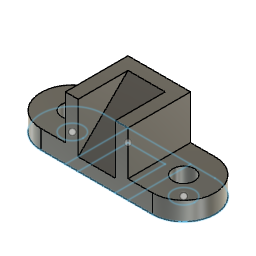
A2 (Autodesk Fusion 360 design; units mm, degrees)
Autodesk Fusion 360 part; units mm, degrees
sketch "Sketch1" plane through (0, 0, 0) normal (0, 0, 1) x (1, 0, 0)
  circle A0 centre (-57, 0.002) radius 11
  circle A1 centre (57, 0.0006) radius 11
  line L0 (57.0004, 32.0006) -> (-56.9996, 32.002)
  line L1 (-57.0004, -31.998) -> (56.9996, -31.9994)
  line L2 (-32, 32.0017) -> (-32.0007, -31.9983)
  line L3 (32.0004, 32.0009) -> (31.9996, -31.9991)
  line L4 (-19.0007, -31.9985) -> (-19.0002, 19.0015)
  line L5 (18.9996, -31.9989) -> (19.0002, 19.0011)
  line L6 (-19.0004, 19.0015) -> (19.0002, 19.0011)
  arc A2 (-56.9996, 32.002) -> (-57.0004, -31.998) centre (-57, 0.002) ccw
  arc A3 (56.9996, -31.9994) -> (57.0004, 32.0006) centre (57, 0.0006) ccw
  dimension "d1" = 22
  dimension "d2" = 57
  dimension "d3" = 22
  dimension "d4" = 57
  dimension "d7" = 114
  dimension "d8" = 64
  dimension "d9" = 32
  dimension "d10" = 32
  dimension "d13" = 51
  constraint tangent L0 A2
  constraint tangent L0 A3
  constraint tangent L1 A3
  constraint tangent L1 A2
  constraint coincident L1 L2.end
  constraint perpendicular L1 L2
  constraint coincident L0 L3.start
  constraint coincident L1 L3.end
  constraint perpendicular L1 L3
  constraint perpendicular L0 L4
  constraint perpendicular L0 L5
  constraint perpendicular L5 L6
  constraint coincident L6 L4.end
  constraint concentric A0 A2
  constraint concentric A1 A3
  constraint perpendicular L0 L2
  constraint coincident L0 L2.start
  constraint coincident L1 L4.start
  constraint coincident L1 L5.start
  measures "d1" diameter of A0
  measures "d2" horizontal distance of origin A0.centre
  measures "d3" diameter of A1
  measures "d4" distance of origin A1.centre
  measures "d7" horizontal distance of L0.start L0.end
  measures "d8" vertical distance of L0.end L1.start
  measures "d9" horizontal distance of origin L2.start
  measures "d10" distance of origin L3
  measures "d13" vertical distance of L4.start L6.start
extrude "Extrude2" add sketch "Sketch1" along normal blind 19 contours L0 L1 L3 A3 makes body 1
extrude "Extrude1" add sketch "Sketch1" along normal blind 19 separate body contours L0 L1 L2 A2 makes body 2
extrude "Extrude3" add sketch "Sketch1" along normal blind 13 separate body contours L1 L4 L5 L6 makes body 3
extrude "Extrude4" add sketch "Sketch1" along normal blind 64 contours L0 L1 L2 L3 L4 L5 L6 bodies 1 2 3
sketch "Sketch3" plane through (19, -0.0002, 0) normal (-1, 0.000012, 0) x (-0.000012, -1, 0)
  line L0 (-19.0013, 13) -> (31.9987, 13)
  line L1 (31.9987, 13) -> (31.9987, 64)
  line L2 (31.9987, 64) -> (-19.0013, 64)
  line L3 (-19.0013, 64) -> (-19.0013, 13)
  line L4 (-19.0013, 64) -> (31.9987, 13)
  line L5 (-19.0013, 64) -> (-19.0013, 13)
  line L6 (31.9987, 13) -> (-19.0013, 13)
  constraint coincident L2.end L3.start
  constraint coincident L0.end L1.start
  constraint coincident L0.start L3.end
extrude "Extrude5" add sketch "Sketch3" along normal blind 38 contours L0 L3 L4 L5 L6 bodies 1
